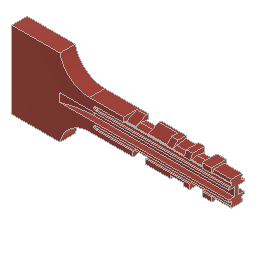
sentry (Autodesk Fusion 360 design; units mm, degrees)
Autodesk Fusion 360 part; units mm, degrees
sketch "base" plane through (0, 0, 0) normal (1, 0, 0) x (0, 1, 0)
  line L0 (0, 0) -> (0, 2.2125)
  line L1 (0, 0) -> (3.2, 0)
  line L2 (0, 2.2125) -> (1.175, 2.2125)
  line L3 (1.175, 2.2125) -> (1.175, 3.9625)
  line L4 (1.175, 3.9625) -> (0, 3.9625)
  line L5 (0, 3.9625) -> (0, 6.175)
  line L6 (0, 6.175) -> (3.2, 6.175)
  line L7 (3.2, 6.175) -> (3.2, 3.9625)
  line L8 (3.2, 3.9625) -> (2.025, 3.9625)
  line L9 (2.025, 3.9625) -> (2.025, 2.2125)
  line L10 (2.025, 2.2125) -> (3.2, 2.2125)
  line L11 (3.2, 2.2125) -> (3.2, 0)
  dimension "d1" = 2.2125
  dimension "d2" = 3.2
  dimension "d3" = 1.175
  dimension "d4" = 1.75
  dimension "d5" = 1.175
  dimension "d6" = 2.2125
  dimension "d7" = 3.2
  dimension "d8" = 2.2125
  dimension "d9" = 1.175
  dimension "d10" = 1.75
  dimension "d11" = 1.175
  constraint coincident L0.start L1.start
  constraint vertical L0
  constraint perpendicular L0 L1
  constraint perpendicular L0 L2
  constraint perpendicular L2 L3
  constraint perpendicular L3 L4
  constraint perpendicular L4 L5
  constraint perpendicular L5 L6
  constraint perpendicular L6 L7
  constraint perpendicular L7 L8
  constraint perpendicular L8 L9
  constraint perpendicular L9 L10
  measures "d1" distance of L0.start L0.end
  measures "d2" distance of L0.start L1.end
  measures "d3" distance of L0.end L2.end
  measures "d4" distance of L2.end L3.end
  measures "d5" distance of L3.end L4.end
  measures "d6" distance of L4.end L5.end
  measures "d7" distance of L5.end L6.end
  measures "d8" distance of L6.end L7.end
  measures "d9" distance of L7.end L8.end
  measures "d10" distance of L8.end L9.end
  measures "d11" distance of L9.end L10.end
extrude "Extrude1" add sketch "base" against normal blind 35
sketch "warding" plane through (0, 0, 0) normal (1, 0, 0) x (0, 1, 0)
  line L0 (0, 0) -> (3.2, 0) construction
  line L1 (0, 0) -> (0, 6.175) construction
  line L2 (0, 6.175) -> (3.2, 6.175) construction
  line L3 (0, 0) -> (0, 1) construction
  line L4 (3.2, 0) -> (3.2, 1) construction
  line L5 (0, 6.175) -> (0, 5.175) construction
  line L6 (3.2, 6.175) -> (3.2, 5.175) construction
  line L7 (0, 1) -> (0.6, 1)
  line L8 (3.2, 1) -> (2.6, 1)
  line L9 (0, 5.175) -> (0.6, 5.175)
  line L10 (3.2, 5.175) -> (2.6, 5.175)
  line L11 (0.6, 1) -> (0.6, 1.75)
  line L12 (2.6, 1) -> (2.6, 1.75)
  line L13 (0.6, 5.175) -> (0.6, 4.425)
  line L14 (2.6, 5.175) -> (2.6, 4.425)
  line L15 (0, 1) -> (0, 1.75)
  line L16 (3.2, 1) -> (3.2, 1.75)
  line L17 (0, 5.175) -> (0, 4.425)
  line L18 (3.2, 5.175) -> (3.2, 4.425)
  line L19 (0.6, 1.75) -> (0, 1.75)
  line L20 (3.2, 1.75) -> (2.6, 1.75)
  line L21 (0.6, 4.425) -> (0, 4.425)
  line L22 (2.6, 4.425) -> (3.2, 4.425)
  dimension "d14" = 3.2
  dimension "d15" = 6.175
  dimension "d16" = 3.2
  dimension "d17" = 1
  dimension "d18" = 1
  dimension "d19" = 1
  dimension "d20" = 1
  dimension "d21" = 0.6
  dimension "d22" = 0.6
  dimension "d23" = 0.6
  dimension "d24" = 0.6
  dimension "d25" = 0.75
  dimension "d26" = 0.75
  dimension "d27" = 0.75
  dimension "d28" = 0.75
  dimension "d29" = 0.75
  dimension "d30" = 0.75
  dimension "d31" = 0.75
  dimension "d32" = 0.75
  constraint coincident L0.start L1.start
  constraint horizontal L0
  constraint perpendicular L0 L1
  constraint perpendicular L1 L2
  constraint perpendicular L0 L3
  constraint perpendicular L0 L4
  constraint perpendicular L2 L5
  constraint perpendicular L2 L6
  constraint perpendicular L3 L7
  constraint perpendicular L4 L8
  constraint perpendicular L5 L9
  constraint perpendicular L6 L10
  constraint perpendicular L7 L11
  constraint perpendicular L8 L12
  constraint perpendicular L9 L13
  constraint perpendicular L10 L14
  constraint perpendicular L7 L15
  constraint perpendicular L8 L16
  constraint perpendicular L9 L17
  constraint perpendicular L10 L18
  measures "d14" distance of L0.start L0.end
  measures "d15" distance of L0.start L1.end
  measures "d16" distance of L1.end L2.end
  measures "d17" distance of L0.start L3.end
  measures "d18" distance of L0.end L4.end
  measures "d19" distance of L1.end L5.end
  measures "d20" distance of L2.end L6.end
  measures "d21" distance of L3.end L7.end
  measures "d22" distance of L4.end L8.end
  measures "d23" distance of L5.end L9.end
  measures "d24" distance of L6.end L10.end
  measures "d25" distance of L7.end L11.end
  measures "d26" distance of L8.end L12.end
  measures "d27" distance of L9.end L13.end
  measures "d28" distance of L10.end L14.end
  measures "d29" distance of L3.end L15.end
  measures "d30" distance of L4.end L16.end
  measures "d31" distance of L5.end L17.end
  measures "d32" distance of L6.end L18.end
extrude "Extrude2" cut sketch "warding" against normal blind 28
fillet "Fillet1" radius 0.325 8 edges at (-14, 0.6, 5.175) (-14, 0.6, 1.75) (-14, 0.6, 4.425) (-14, 0.6, 1) (-14, 2.6, 4.425) (-14, 2.6, 1) (-14, 2.6, 5.175) (-14, 2.6, 1.75)
sketch "aws disc" plane through (0, 0, 0) normal (1, 0, 0) x (0, 1, 0)
  line L0 (0, 0) -> (1.6, 0) construction
  line L1 (1.6, 0) -> (1.6, 3.0875) construction
  line L2 (1.6, 3.0875) -> (1.6, 6.175) construction
  line L3 (1.6, 6.175) -> (0, 6.175) construction
  line L4 (1.6, 3.0875) -> (0, 3.0875) construction
  line L5 (1.6, 3.0875) -> (-0.2806, 3.9644) construction
  line L6 (1.6, 3.0875) -> (0, 3.0875) construction
  line L7 (-0.2806, 3.9644) -> (0.7502, 6.175)
  line L8 (1.6, 3.0875) -> (-0.2806, 2.2106) construction
  line L9 (1.6, 3.0875) -> (0, 3.0875) construction
  line L10 (-0.2806, 2.2106) -> (0.7502, 0)
  line L11 (1.6, 3.0875) -> (3.4806, 2.2106) construction
  line L12 (1.6, 3.0875) -> (3.4806, 3.9644) construction
  line L13 (3.4806, 3.9644) -> (2.4498, 6.175)
  line L14 (3.4806, 2.2106) -> (2.4498, 0)
  line L15 (0.7502, 6.175) -> (2.4498, 6.175)
  line L16 (0.7502, 0) -> (2.4498, 0)
  line L17 (-0.2806, 3.9644) -> (-0.2806, 2.2106)
  line L18 (3.4806, 3.9644) -> (3.4806, 2.2106)
  circle A0 centre (1.6, 3.0875) radius 4.25
  dimension "d37" = 1.6
  dimension "d38" = 3.0875
  dimension "d39" = 3.0875
  dimension "d40" = 1.6
  dimension "d41" = 1.6
  dimension "d42" = 25
  dimension "d43" = 2.075
  dimension "d44" = 25
  dimension "d45" = 2.075
  dimension "d46" = 8.5
  constraint coincident L0.start origin
  constraint horizontal L0
  constraint perpendicular L0 L1
  constraint parallel L1 L2
  constraint perpendicular L2 L3
  constraint perpendicular L1 L4
  constraint horizontal L6
  constraint coincident L3 L7.end
  constraint perpendicular L5 L7
  constraint horizontal L9
  constraint perpendicular L8 L10
  constraint equal L7 L10
  constraint parallel L5 L11
  constraint equal L5 L11
  constraint parallel L8 L12
  constraint equal L5 L12
  constraint perpendicular L12 L13
  constraint equal L7 L13
  constraint perpendicular L11 L14
  constraint equal L7 L14
  constraint coincident L1.end L2.start
  measures "d37" distance of L0.start L0.end
  measures "d38" distance of L0.end L1.end
  measures "d39" distance of L1.end L2.end
  measures "d40" distance of L2.end L3.end
  measures "d41" distance of L1.end L4.end
  measures "d42" angle of L5 L6
  measures "d43" distance of L1.end L5.end
  measures "d44" angle of L8 L9
  measures "d45" distance of L1.end L8.end
  measures "d46" diameter of A0
sketch "tip warding" plane through (0, 0, 0) normal (1, 0, 0) x (0, 1, 0)
  line L0 (0, 0) -> (3.2, 0)
  line L1 (1.6, 0) -> (1.6, 6.175) construction
  line L2 (1.6, 6.175) -> (0, 6.175)
  line L3 (1.6, 6.175) -> (3.2, 6.175)
  line L4 (0, 0) -> (0, 0.5)
  line L5 (3.2, 6.175) -> (3.2, 5.675)
  line L6 (0, 0.5) -> (3.2, 0.5)
  line L7 (3.2, 0.5) -> (3.2, 0)
  line L8 (3.2, 5.675) -> (0, 5.675)
  line L9 (0, 5.675) -> (0, 6.175)
  dimension "d47" = 3.2
  dimension "d48" = 6.175
  dimension "d49" = 1.6
  dimension "d50" = 1.6
  dimension "d51" = 0.5
  dimension "d52" = 0.5
  constraint coincident L0.start L4.start
  constraint horizontal L0
  constraint midpoint L0 L1.start
  constraint perpendicular L0 L1
  constraint perpendicular L1 L2
  constraint perpendicular L1 L3
  constraint perpendicular L0 L4
  constraint perpendicular L3 L5
  constraint perpendicular L4 L6
  constraint perpendicular L0 L7
  constraint perpendicular L5 L8
  constraint perpendicular L2 L9
  measures "d47" distance of L0.start L0.end
  measures "d48" distance of L1.start L1.end
  measures "d49" distance of L1.end L2.end
  measures "d50" distance of L1.end L3.end
  measures "d51" distance of L0.start L4.end
  measures "d52" distance of L3.end L5.end
extrude "Extrude3" cut sketch "tip warding" against normal blind 3.62
extrude "Extrude4" cut sketch "aws disc" against normal blind 3.62
sketch "1 cut" plane through (0, 0, 0) normal (1, 0, 0) x (0, 1, 0)
  line L0 (0, 0) -> (1.6, 0) construction
  line L1 (1.6, 0) -> (1.6, 3.0875) construction
  circle A0 centre (1.6, 3.0875) radius 3.65 construction
  line L2 (1.6, 3.0875) -> (3.2484, 6.0612) construction
  line L3 (1.6, 3.0875) -> (5.25, 3.0875) construction
  line L4 (1.6, 3.0875) -> (-0.0484, 0.1138) construction
  line L5 (3.2484, 6.0612) -> (2.0872, 6.7048)
  line L6 (3.2484, 6.0612) -> (4.4095, 5.4176)
  line L7 (-0.0484, 0.1138) -> (1.1128, -0.5298)
  line L8 (-0.0484, 0.1138) -> (-1.2095, 0.7574)
  circle A1 centre (1.6, 3.0875) radius 4.25
  arc A2 (2.0872, 6.7048) -> (-1.2095, 0.7574) centre (1.6, 3.0875) ccw
  arc A3 (1.1128, -0.5298) -> (4.4095, 5.4176) centre (1.6, 3.0875) ccw
  dimension "d57" = 1.6
  dimension "d58" = 3.0875
  dimension "d59" = 7.3
  dimension "d60" = 61
  dimension "d61" = 3.4
  dimension "d62" = 8.5
  dimension "d63" = 3.65
  dimension "d64" = 3.65
  constraint coincident L0.start origin
  constraint horizontal L0
  constraint perpendicular L0 L1
  constraint coincident L1.end A0.centre
  constraint horizontal L3
  constraint coincident A0 L3.end
  constraint parallel L2 L4
  constraint equal L2 L4
  constraint coincident A0 L5.end
  constraint perpendicular L2 L5
  constraint coincident A0 L6.end
  constraint perpendicular L2 L6
  constraint coincident A0 L7.end
  constraint perpendicular L4 L7
  constraint coincident A0 L8.end
  constraint perpendicular L4 L8
  constraint concentric A0 A1
  measures "d57" distance of L0.start L0.end
  measures "d58" distance of L0.end L1.end
  measures "d59" diameter of A0
  measures "d60" angle of L2 L3
  measures "d61" distance of L1.end L2.end
  measures "d62" diameter of A1
  measures "d63" radius of A2
  measures "d64" radius of A3
sketch "2 cut" plane through (0, 0, 0) normal (1, 0, 0) x (0, 1, 0)
  line L0 (0, 0) -> (1.6, 0) construction
  line L1 (1.6, 0) -> (1.6, 3.0875) construction
  line L2 (1.6, 3.0875) -> (-0.4087, 4.1555) construction
  line L3 (1.6, 3.0875) -> (-1.9691, 3.0875) construction
  line L4 (1.6, 3.0875) -> (3.6087, 2.0195) construction
  line L5 (-0.4087, 4.1555) -> (0.8823, 6.5837)
  line L6 (3.6087, 2.0195) -> (2.3177, -0.4087)
  circle A0 centre (1.6, 3.0875) radius 3.5691 construction
  line L7 (3.6087, 2.0195) -> (3.6087, 6.0376)
  line L8 (-0.4087, 4.1555) -> (-0.4087, 0.1374)
  arc A1 (3.6087, 6.0376) -> (0.8823, 6.5837) centre (1.6, 3.0875) ccw
  arc A2 (-0.4087, 0.1374) -> (2.3177, -0.4087) centre (1.6, 3.0875) ccw
  circle A3 centre (1.6, 3.0875) radius 4.25
  dimension "d65" = 1.6
  dimension "d66" = 3.0875
  dimension "d67" = 28
  dimension "d68" = 2.275
  dimension "d69" = 2.275
  dimension "d70" = 2.75
  dimension "d71" = 2.75
  dimension "d72" = 3.5691
  dimension "d73" = 3.5691
  dimension "d74" = 8.5
  constraint coincident L0.start origin
  constraint horizontal L0
  constraint perpendicular L0 L1
  constraint horizontal L3
  constraint parallel L2 L4
  constraint perpendicular L2 L5
  constraint perpendicular L4 L6
  constraint coincident L1.end L2.start
  constraint coincident L5.end A0
  constraint coincident L3.end A0
  constraint coincident A0 L7.end
  constraint vertical L7
  constraint coincident A0 L8.end
  constraint parallel L7 L8
  constraint concentric A2 A3
  measures "d65" distance of L0.start L0.end
  measures "d66" distance of L0.end L1.end
  measures "d67" angle of L2 L3
  measures "d68" distance of L1.end L2.end
  measures "d69" distance of L1.end L4.end
  measures "d70" distance of L2.end L5.end
  measures "d71" distance of L4.end L6.end
  measures "d72" radius of A2
  measures "d73" radius of A1
  measures "d74" diameter of A3
sketch "3 cut" plane through (0, 0, 0) normal (1, 0, 0) x (0, 1, 0)
  line L0 (0, 0) -> (1.6, 0) construction
  line L1 (1.6, 0) -> (1.6, 3.0875) construction
  line L2 (1.6, 3.0875) -> (0.0197, 4.724) construction
  line L3 (1.6, 3.0875) -> (-0.675, 3.0875) construction
  line L4 (1.6, 3.0875) -> (3.1803, 1.451) construction
  line L5 (0.0197, 4.724) -> (1.9978, 6.6343)
  line L6 (3.1803, 1.451) -> (1.2022, -0.4593)
  line L7 (1.6, 3.0875) -> (-0.675, 3.0875) construction
  line L8 (1.6, 3.0875) -> (3.875, 3.0875) construction
  circle A0 centre (1.6, 3.0875) radius 3.5691 construction
  arc A1 (0.0197, 4.724) -> (-0.675, 3.0875) centre (1.6, 3.0875) ccw
  arc A2 (3.1803, 1.451) -> (3.875, 3.0875) centre (1.6, 3.0875) ccw
  line L9 (3.875, 3.0875) -> (3.875, 5.8375)
  line L10 (-0.675, 3.0875) -> (-0.675, 0.3375)
  arc A3 (3.875, 5.8375) -> (1.9978, 6.6343) centre (1.6, 3.0875) ccw
  arc A4 (-0.675, 0.3375) -> (1.2022, -0.4593) centre (1.6, 3.0875) ccw
  circle A5 centre (1.6, 3.0875) radius 4.25
  dimension "d75" = 1.6
  dimension "d76" = 3.0875
  dimension "d77" = 46
  dimension "d78" = 2.275
  dimension "d79" = 2.275
  dimension "d80" = 2.75
  dimension "d81" = 2.75
  dimension "d82" = 2.275
  dimension "d83" = 2.275
  dimension "d84" = 2.275
  dimension "d85" = 2.275
  dimension "d86" = 3.5691
  dimension "d87" = 3.5691
  dimension "d88" = 8.5
  constraint coincident L0.start origin
  constraint horizontal L0
  constraint perpendicular L0 L1
  constraint horizontal L3
  constraint parallel L2 L4
  constraint perpendicular L2 L5
  constraint perpendicular L4 L6
  constraint perpendicular L1 L7
  constraint perpendicular L1 L8
  constraint coincident L1.end L2.start
  constraint coincident L5.end A0
  constraint coincident A0 L9.end
  constraint tangent A2 L9
  constraint coincident A0 L10.end
  constraint tangent A1 L10
  constraint concentric A4 A5
  measures "d75" distance of L0.start L0.end
  measures "d76" distance of L0.end L1.end
  measures "d77" angle of L2 L3
  measures "d78" distance of L1.end L2.end
  measures "d79" distance of L1.end L4.end
  measures "d80" distance of L2.end L5.end
  measures "d81" distance of L4.end L6.end
  measures "d82" distance of L1.end L3.end
  measures "d83" distance of L1.end L8.end
  measures "d84" radius of A1
  measures "d85" radius of A2
  measures "d86" radius of A4
  measures "d87" radius of A3
  measures "d88" diameter of A5
sketch "4 cut" plane through (0, 0, 0) normal (1, 0, 0) x (0, 1, 0)
  line L0 (0, 0) -> (1.6, 0) construction
  line L1 (1.6, 0) -> (1.6, 3.0875) construction
  line L2 (1.6, 3.0875) -> (0.6027, 5.1323) construction
  line L3 (1.6, 3.0875) -> (-0.675, 3.0875) construction
  line L4 (1.6, 3.0875) -> (2.5973, 1.0427) construction
  line L5 (0.6027, 5.1323) -> (3.0744, 6.3378)
  line L6 (2.5973, 1.0427) -> (0.1256, -0.1628)
  line L7 (1.6, 3.0875) -> (-0.675, 3.0875) construction
  line L8 (1.6, 3.0875) -> (3.875, 3.0875) construction
  arc A0 (0.6027, 5.1323) -> (-0.675, 3.0875) centre (1.6, 3.0875) ccw
  arc A1 (2.5973, 1.0427) -> (3.875, 3.0875) centre (1.6, 3.0875) ccw
  circle A2 centre (1.6, 3.0875) radius 3.5691 construction
  line L9 (3.875, 3.0875) -> (3.875, 5.8375)
  line L10 (-0.675, 3.0875) -> (-0.675, 0.3375)
  arc A3 (3.875, 5.8375) -> (3.0744, 6.3378) centre (1.6, 3.0875) ccw
  arc A4 (-0.675, 0.3375) -> (0.1256, -0.1628) centre (1.6, 3.0875) ccw
  circle A5 centre (1.6, 3.0875) radius 4.25
  dimension "d89" = 1.6
  dimension "d90" = 3.0875
  dimension "d91" = 64
  dimension "d92" = 2.275
  dimension "d93" = 2.275
  dimension "d94" = 2.75
  dimension "d95" = 2.75
  dimension "d96" = 2.275
  dimension "d97" = 2.275
  dimension "d98" = 2.275
  dimension "d99" = 2.275
  dimension "d100" = 3.5691
  dimension "d101" = 3.5691
  dimension "d102" = 8.5
  constraint coincident L0.start origin
  constraint horizontal L0
  constraint perpendicular L0 L1
  constraint horizontal L3
  constraint parallel L2 L4
  constraint perpendicular L2 L5
  constraint perpendicular L4 L6
  constraint perpendicular L1 L7
  constraint perpendicular L1 L8
  constraint concentric A1 A2
  constraint coincident L5.end A2
  constraint coincident A2 L9.end
  constraint tangent A1 L9
  constraint coincident A2 L10.end
  constraint tangent A0 L10
  constraint concentric A2 A5
  measures "d89" distance of L0.start L0.end
  measures "d90" distance of L0.end L1.end
  measures "d91" angle of L2 L3
  measures "d92" distance of L1.end L2.end
  measures "d93" distance of L1.end L4.end
  measures "d94" distance of L2.end L5.end
  measures "d95" distance of L4.end L6.end
  measures "d96" distance of L1.end L3.end
  measures "d97" distance of L1.end L8.end
  measures "d98" radius of A0
  measures "d99" radius of A1
  measures "d100" radius of A4
  measures "d101" radius of A3
  measures "d102" diameter of A5
sketch "5 cut" plane through (0, 0, 0) normal (1, 0, 0) x (0, 1, 0)
  line L0 (0, 0) -> (1.6, 0) construction
  line L1 (1.6, 0) -> (1.6, 3.0875) construction
  line L2 (1.6, 3.0875) -> (1.2834, 5.3404) construction
  line L3 (1.6, 3.0875) -> (-0.675, 3.0875) construction
  line L4 (1.6, 3.0875) -> (1.9166, 0.8346) construction
  line L5 (1.2834, 5.3404) -> (4.0066, 5.7231)
  line L6 (1.9166, 0.8346) -> (-0.8066, 0.4519)
  line L7 (1.6, 3.0875) -> (-0.675, 3.0875) construction
  line L8 (1.6, 3.0875) -> (3.875, 3.0875) construction
  arc A0 (1.2834, 5.3404) -> (-0.675, 3.0875) centre (1.6, 3.0875) ccw
  arc A1 (1.9166, 0.8346) -> (3.875, 3.0875) centre (1.6, 3.0875) ccw
  circle A2 centre (1.6, 3.0875) radius 3.5691 construction
  line L9 (3.875, 3.0875) -> (4.0066, 5.7231)
  line L10 (-0.8066, 0.4519) -> (-0.675, 3.0875)
  circle A3 centre (1.6, 3.0875) radius 4.25
  dimension "d103" = 1.6
  dimension "d104" = 3.0875
  dimension "d105" = 82
  dimension "d106" = 2.275
  dimension "d107" = 2.275
  dimension "d108" = 2.75
  dimension "d109" = 2.75
  dimension "d110" = 2.275
  dimension "d111" = 2.275
  dimension "d112" = 2.275
  dimension "d113" = 2.275
  dimension "d114" = 8.5
  constraint coincident L0.start origin
  constraint horizontal L0
  constraint perpendicular L0 L1
  constraint horizontal L3
  constraint parallel L2 L4
  constraint perpendicular L2 L5
  constraint perpendicular L4 L6
  constraint perpendicular L1 L7
  constraint perpendicular L1 L8
  constraint concentric A0 A2
  constraint coincident L5.end A2
  constraint concentric A0 A3
  measures "d103" distance of L0.start L0.end
  measures "d104" distance of L0.end L1.end
  measures "d105" angle of L2 L3
  measures "d106" distance of L1.end L2.end
  measures "d107" distance of L1.end L4.end
  measures "d108" distance of L2.end L5.end
  measures "d109" distance of L4.end L6.end
  measures "d110" distance of L1.end L3.end
  measures "d111" distance of L1.end L8.end
  measures "d112" radius of A0
  measures "d113" radius of A1
  measures "d114" diameter of A3
sketch "6 cut" plane through (0, 0, 0) normal (1, 0, 0) x (0, 1, 0)
  line L0 (0, 0) -> (1.6, 0) construction
  line L1 (1.6, 0) -> (1.6, 3.0875) construction
  line L2 (1.6, 3.0875) -> (1.6, 5.3625) construction
  line L3 (1.6, 3.0875) -> (1.6, 0.8125) construction
  line L4 (1.6, 5.3625) -> (4.3082, 4.885)
  line L5 (1.6, 0.8125) -> (-1.1082, 1.29)
  line L6 (1.6, 3.0875) -> (-0.675, 3.0875) construction
  line L7 (1.6, 3.0875) -> (3.875, 3.0875) construction
  arc A0 (1.6, 5.3625) -> (-0.675, 3.0875) centre (1.6, 3.0875) ccw
  arc A1 (1.6, 0.8125) -> (3.875, 3.0875) centre (1.6, 3.0875) ccw
  circle A2 centre (1.6, 3.0875) radius 3.2504 construction
  line L8 (3.875, 3.0875) -> (4.3082, 4.885)
  line L9 (-1.1082, 1.29) -> (-0.675, 3.0875)
  circle A3 centre (1.6, 3.0875) radius 4.25
  dimension "d115" = 1.6
  dimension "d116" = 3.0875
  dimension "d117" = 2.275
  dimension "d118" = 2.275
  dimension "d119" = 2.75
  dimension "d120" = 2.75
  dimension "d121" = 2.275
  dimension "d122" = 2.275
  dimension "d123" = 2.275
  dimension "d124" = 2.275
  dimension "d125" = 8.5
  dimension "d156" = 80
  dimension "d157" = 80
  constraint coincident L0.start origin
  constraint horizontal L0
  constraint perpendicular L0 L1
  constraint parallel L1 L2
  constraint parallel L1 L3
  constraint perpendicular L3 L6
  constraint perpendicular L2 L7
  constraint coincident L1.end L2.start
  constraint coincident L4.end A2
  constraint concentric A1 A3
  measures "d115" distance of L0.start L0.end
  measures "d116" distance of L0.end L1.end
  measures "d117" distance of L1.end L2.end
  measures "d118" distance of L1.end L3.end
  measures "d119" distance of L2.end L4.end
  measures "d120" distance of L3.end L5.end
  measures "d121" distance of L1.end L6.end
  measures "d122" distance of L1.end L7.end
  measures "d123" radius of A0
  measures "d124" radius of A1
  measures "d125" diameter of A3
  measures "d156" angle of L2 L4
  measures "d157" angle of L3 L5
extrude "1" cut sketch "1 cut" along normal mid plane 2.6 from surface at -4.92
extrude "2" cut sketch "6 cut" along normal mid plane 2.6 from surface at -6.87
extrude "3" cut sketch "2 cut" along normal mid plane 2.6 from surface at -8.82
extrude "4" cut sketch "5 cut" along normal mid plane 2.6 from surface at -10.77
extrude "5" cut sketch "3 cut" along normal mid plane 2.6 from surface at -12.72
extrude "6" cut sketch "4 cut" along normal mid plane 2.6 from surface at -14.67
extrude "7" cut sketch "4 cut" along normal mid plane 2.6 from surface at -16.62
extrude "8" cut sketch "6 cut" along normal mid plane 2.6 from surface at -18.57
extrude "9" cut sketch "4 cut" along normal mid plane 2.6 from surface at -20.52
fillet "Fillet2" radius 0.35 20 edges at (-28, 0.1375, 4.425) (-28, 0.5048, 4.5202) (-28, 0.6, 4.8) (-28, 0.5048, 5.0798) (-28, 0.1375, 5.175) (-28, 0.1375, 1) (-28, 0.5048, 1.0952) (-28, 0.6, 1.375) (-28, 0.5048, 1.6548) (-28, 0.1375, 1.75) (-28, 3.0625, 4.425) (-28, 2.6952, 4.5202) (-28, 2.6, 4.8) (-28, 2.6952, 5.0798) (-28, 3.0625, 5.175) (-28, 3.0625, 1) (-28, 2.6952, 1.0952) (-28, 2.6, 1.375) (-28, 2.6952, 1.6548) (-28, 3.0625, 1.75)
sketch "Sketch11" plane through (-35, 0, 0) normal (-1, 0, 0) x (0, -1, 0)
  line L0 (-3.2, 0) -> (0, 0)
  line L1 (0, 0) -> (0, 2.2125)
  line L2 (0, 2.2125) -> (-1.175, 2.2125)
  line L3 (-1.175, 2.2125) -> (-1.175, 3.9625)
  line L4 (-1.175, 3.9625) -> (0, 3.9625)
  line L5 (0, 3.9625) -> (0, 6.175)
  line L6 (0, 6.175) -> (-3.2, 6.175)
  line L7 (-3.2, 6.175) -> (-3.2, 3.9625)
  line L8 (-3.2, 3.9625) -> (-2.025, 3.9625)
  line L9 (-2.025, 3.9625) -> (-2.025, 2.2125)
  line L10 (-2.025, 2.2125) -> (-3.2, 2.2125)
  line L11 (-3.2, 2.2125) -> (-3.2, 0)
  line L12 (0, 0) -> (0, 6.175) construction
  line L13 (0, 3.0875) -> (0, 11.0875)
  line L14 (0, 11.0875) -> (-3.2, 11.0875)
  line L15 (-3.2, 11.0875) -> (-3.2, -4.9125)
  line L16 (-3.2, -4.9125) -> (0, -4.9125)
  line L17 (0, -4.9125) -> (0, 6.175)
  dimension "d160" = 8
  dimension "d161" = 3.2
  dimension "d162" = 16
  dimension "d163" = 3.2
  constraint coincident L0.end L1.start
  constraint coincident L5.end L6.start
  constraint midpoint L12 L13.start
  constraint perpendicular L6 L13
  constraint perpendicular L13 L14
  constraint perpendicular L14 L15
  constraint perpendicular L15 L16
  measures "d160" distance of L13.start L13.end
  measures "d161" distance of L13.end L14.end
  measures "d162" distance of L14.end L15.end
  measures "d163" distance of L15.end L16.end
extrude "Extrude14" add sketch "Sketch11" along normal blind 10
fillet "Fillet3" radius 6.25 2 edges at (-35, 1.6, 0) (-35, 1.6, 6.175)
fillet "Fillet4" radius 16.25 2 edges at (-35, 1.175, 3.0875) (-35, 2.025, 3.0875)
equation "d5 = d3"
equation "d6 = d1"
equation "d7 = d2"
equation "d8 = d1"
equation "d9 = d3"
equation "d10 = d4"
equation "d11 = d3"
equation "d14 = d2"
equation "d15 = d1 * 2 + d4"
equation "d16 = d2"
equation "d18 = d17"
equation "d19 = d17"
equation "d20 = d17"
equation "d22 = d21"
equation "d23 = d21"
equation "d24 = d21"
equation "d26 = d25"
equation "d27 = d25"
equation "d28 = d25"
equation "d29 = d25"
equation "d30 = d25"
equation "d31 = d25"
equation "d32 = d25"
equation "d37 = d2 / 2"
equation "d38 = d1 + d4 / 2"
equation "d39 = d38"
equation "d40 = d37"
equation "d41 = d37"
equation "d43 = ( 4.15 / 2 ) * 1 mm"
equation "d44 = d42"
equation "d45 = d43"
equation "d47 = d2"
equation "d48 = d1 * 2 + d4"
equation "d49 = d2 / 2"
equation "d50 = d49"
equation "d52 = d51"
equation "d53 = -3.62 mm"
equation "d55 = d53"
equation "d57 = d2 / 2"
equation "d58 = d1 + 0.5 * d4"
equation "d65 = d2 / 2"
equation "d66 = d1 + d4 / 2"
equation "d68 = ( 4.55 / 2 ) * 1 mm"
equation "d69 = d68"
equation "d71 = d70"
equation "d75 = d2 / 2"
equation "d76 = d1 + d4 / 2"
equation "d78 = d68"
equation "d79 = d68"
equation "d80 = d70"
equation "d81 = d70"
equation "d82 = d68"
equation "d83 = d68"
equation "d89 = d2 / 2"
equation "d90 = d1 + d4 / 2"
equation "d92 = d68"
equation "d93 = d68"
equation "d94 = d70"
equation "d95 = d70"
equation "d96 = d68"
equation "d97 = d68"
equation "d103 = d2 / 2"
equation "d104 = d1 + d4 / 2"
equation "d106 = d68"
equation "d107 = d68"
equation "d108 = d70"
equation "d109 = d70"
equation "d110 = d68"
equation "d111 = d68"
equation "d115 = d2 / 2"
equation "d116 = d1 + d4 / 2"
equation "d117 = d68"
equation "d118 = d68"
equation "d119 = d70"
equation "d120 = d70"
equation "d121 = d68"
equation "d122 = d68"
equation "offset = 3.62 mm - 0.65 mm"
equation "spacing = 1.95 mm"
equation "width = 1.3 mm"
equation "d129 = -offset - ( spacing * 1 )"
equation "d130 = width"
equation "d132 = -offset - ( spacing * 2 )"
equation "d133 = width"
equation "d135 = -offset - ( spacing * 3 )"
equation "d136 = width"
equation "d138 = -offset - ( spacing * 4 )"
equation "d139 = width"
equation "d141 = -offset - ( spacing * 5 )"
equation "d142 = width"
equation "d144 = -offset - ( spacing * 6 )"
equation "d145 = width"
equation "d147 = -offset - ( spacing * 7 )"
equation "d148 = width"
equation "d150 = -offset - ( spacing * 8 )"
equation "d151 = width"
equation "d153 = -offset - ( spacing * 9 )"
equation "d154 = width"
equation "d157 = d156"
equation "d161 = d2"
equation "d162 = d160 * 2"
equation "d163 = d161"
named bodies: "key"
